Autodesk Fusion 360 part; units mm, degrees
(part 2 of 2)
extrude "Extrude1" add sketch "Sketch1" along normal blind 6.35 contours L0 L3 L21 L247 | L0 L1 L2 L3 L4 L5 L6 L7 L8 L9 L10 L11 L12 L13 L14 L15 L16 L17 L18 L19 L20 L21 L22 L35 L36 L49 L50 L63 L64 L77 L78 L91 L92 L105 L106 L119 L120 L131 L134 L147 L148 L161 L162 L177 L178 L191 L192 L193 L194 L197 L198 L201 L202 L205 L206 L209 L210 L213 L214 L217 L218 L219 L220 L221 L222 L223 L224 L225 L227 L228 L229 L230 L231 L232 L233 L234 L235 L236 L237 L238 L239 L240 L241 L242 L243 L244 L245 L246 L247 L248 L251 L276 L277 L299 L300 L303 L305 L318 L353 L356 L357 L358 L359 L362 L366 L368 L371 L376 L377 L380 L381 L386 L387 L392 L393 L398 L399 L404 L405 L410 L411 L412 L421 L422 L427 L428 L431 L432 L435 L436 | L0 L22 L246 L248 | L3 L19 L20 L251 | L0 L49 L244 L245 | L3 L17 L18 L299 | L0 L50 L242 L243 | L3 L14 L16 L300 | L0 L77 L240 L241 | L3 L13 L15 L353 | L0 L78 L238 L239 | L3 L11 L12 L358 | L0 L105 L236 L237 | L3 L9 L10 L359 | L0 L106 L234 L235 | L2 L3 L8 L356 | L0 L131 L232 L233 | L2 L35 L357 L362 | L0 L147 L230 L231 | L2 L36 L366 L368 | L0 L148 L228 L229 | L2 L63 L371 L376 | L0 L177 L225 L227 | L2 L64 L377 L380 | L0 L178 L223 L224 | L2 L91 L381 L387 | L0 L219 L221 L222 | L2 L92 L386 L392 | L0 L1 L218 L220 | L2 L119 L393 L398 | L1 L214 L217 L276 | L2 L120 L399 L405 | L1 L210 L213 L277 | L2 L134 L318 L404 | L1 L206 L209 L303 | L2 L161 L410 L411 | L1 L202 L205 L305 | L2 L162 L412 L421 | L1 L198 L201 L436 | L2 L191 L422 L427 | L1 L194 L197 L435 | L2 L192 L428 L431 | L1 L2 L193 L432 | L23 L24 L249 L250 | L25 L26 L298 L302 | L27 L28 L350 L355 | L29 L30 L351 L354 | L31 L32 L361 L363 | L33 L34 L360 L364 | L37 L38 L367 L370 | L39 L40 L365 L369 | L41 L42 L346 L352 | L43 L44 L345 L349 | L45 L46 L297 L301 | L47 L48 L252 L297 | L51 L52 L253 L254 | L53 L54 L295 L296 | L55 L56 L343 L348 | L57 L59 L344 L347 | L58 L60 L373 L374 | L61 L62 L372 L375 | L65 L66 L378 L383 | L67 L68 L379 L382 | L69 L70 L339 L341 | L71 L72 L338 L342 | L73 L74 L293 L294 | L75 L76 L255 L259 | L79 L80 L256 L258 | L81 L82 L291 L292 | L83 L84 L332 L337 | L85 L86 L333 L340 | L87 L88 L385 L388 | L89 L90 L384 L389 | L93 L94 L390 L395 | L95 L96 L391 L394 | L97 L98 L329 L334 | L99 L100 L328 L335 | L101 L102 L261 L290 | L103 L104 L257 L260 | L107 L108 L262 L263 | L109 L110 L288 L289 | L111 L112 L326 L331 | L113 L114 L330 L336 | L115 L116 L397 L402 | L117 L118 L396 L403 | L121 L122 L400 L407 | L123 L124 L401 L406 | L125 L126 L324 L327 | L127 L128 L323 L325 | L129 L133 L286 L287 | L130 L132 L264 L265 | L135 L136 L318 L408 | L137 L138 L318 L409 | L139 L140 L320 L321 | L141 L142 L319 L322 | L143 L144 L284 L285 | L145 L146 L266 L267 | L149 L150 L268 L269 | L151 L152 L282 L283 | L153 L154 L314 L317 | L155 L156 L315 L316 | L157 L158 L415 L418 | L159 L160 L416 L417 | L163 L164 L413 L420 | L165 L166 L414 L419 | L167 L168 L312 L313 | L169 L170 L171 L311 | L172 L183 L184 L306 | L173 L174 L226 L281 | L175 L176 L226 L270 | L179 L180 L272 L273 | L181 L182 L271 L280 | L185 L186 L307 L310 | L187 L188 L424 L425 | L189 L190 L423 L426 | L195 L196 L429 L434 | L199 L200 L430 L433 | L203 L204 L304 L308 | L207 L208 L304 L309 | L211 L212 L278 L279 | L215 L216 L274 L275
extrude "Extrude2" cut sketch "Sketch1" against normal blind 0.7874 from surface at 6.35 contours L0 L1 L2 L3 L4 L5 L6 L7 L8 L9 L10 L11 L12 L13 L14 L15 L16 L17 L18 L19 L20 L21 L22 L35 L36 L49 L50 L63 L64 L77 L78 L91 L92 L105 L106 L119 L120 L131 L134 L147 L148 L161 L162 L177 L178 L191 L192 L193 L194 L197 L198 L201 L202 L205 L206 L209 L210 L213 L214 L217 L218 L219 L220 L221 L222 L223 L224 L225 L227 L228 L229 L230 L231 L232 L233 L234 L235 L236 L237 L238 L239 L240 L241 L242 L243 L244 L245 L246 L247 L248 L251 L276 L277 L299 L300 L303 L305 L318 L353 L356 L357 L358 L359 L362 L366 L368 L371 L376 L377 L380 L381 L386 L387 L392 L393 L398 L399 L404 L405 L410 L411 L412 L421 L422 L427 L428 L431 L432 L435 L436
hole "Hole1" at (12.7, 0, 12.7) direction (0, 1, 0) diameter 12.7 end through all
hole "Hole2" at (57.15, 0, 12.7) direction (0, 1, 0) diameter 12.7 depth 6.35 tip angle 118
